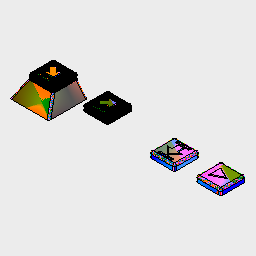
keycaps_debugsymbols_v2 (Autodesk Fusion 360 design; units mm, degrees)
Autodesk Fusion 360 part; units mm, degrees
note: some values were not read from the file. Chosen so that the rebuilt part matches the saved one: which sketch regions a step uses; that a step has no effect.
mesh "Netz1" [no effect]
sketch "Skizze1" plane through (5.433, 7.5669, 0.0261) normal (0, 0, 1) x (1, 0, 0)
  line L0 (-3.1492, -9.717) -> (-7.3992, -9.717) construction
  line L1 (-7.3992, -9.717) -> (-7.3992, -5.467) construction
  line L2 (-7.3992, -5.467) -> (-3.1492, -5.467) construction
  line L3 (-3.1492, -5.467) -> (-3.1492, -9.717) construction
  line L4 (-3.1492, -9.717) -> (-7.3992, -5.467) construction
  line L5 (-7.3992, -9.717) -> (-3.1492, -5.467) construction
  circle A0 centre (-5.2742, -7.592) radius 3.0052
  line L6 (-4.6092, -5.467) -> (-5.9392, -5.467)
  line L7 (-5.9392, -9.717) -> (-4.6092, -9.717)
  line L8 (-4.6092, -5.467) -> (-5.9392, -9.717) construction
  line L9 (-5.9392, -5.467) -> (-4.6092, -9.717) construction
  line L10 (-7.3992, -8.337) -> (-7.3992, -6.847)
  line L11 (-3.1492, -6.847) -> (-3.1492, -8.337)
  line L12 (-3.1492, -8.337) -> (-7.3992, -6.847) construction
  line L13 (-7.3992, -8.337) -> (-3.1492, -6.847) construction
  line L14 (-5.9392, -5.467) -> (-5.9392, -6.847)
  line L15 (-5.9392, -8.337) -> (-5.9392, -9.717)
  line L16 (-3.1492, -8.337) -> (-4.6092, -8.337)
  line L17 (-5.9392, -8.337) -> (-7.3992, -8.337)
  line L18 (-4.6092, -9.717) -> (-4.6092, -8.337)
  line L19 (-4.6092, -6.847) -> (-4.6092, -5.467)
  line L20 (-7.3992, -6.847) -> (-5.9392, -6.847)
  line L21 (-4.6092, -6.847) -> (-3.1492, -6.847)
  line L22 (3.0758, 0.758) -> (-13.6242, 0.758)
  line L23 (-13.6242, 0.758) -> (-13.6242, -15.942)
  line L24 (-13.6242, -15.942) -> (3.0758, -15.942)
  line L25 (3.0758, -15.942) -> (3.0758, 0.758)
  line L26 (3.0758, 0.758) -> (-13.6242, -15.942) construction
  line L27 (-13.6242, 0.758) -> (3.0758, -15.942) construction
  line L28 (4.0758, -16.942) -> (4.0758, 1.758)
  line L29 (4.0758, 1.758) -> (-14.6242, 1.758)
  line L30 (-14.6242, 1.758) -> (-14.6242, -16.942)
  line L31 (-14.6242, -16.942) -> (4.0758, -16.942)
  point P0 (-5.2742, -7.592)
  point P1 (-5.2742, -7.592)
  point P2 (-5.2742, -7.592)
  point P3 (-5.2742, -7.592)
  dimension "d1" = 4.25
  dimension "d2" = 4.25
  dimension "d3" = 1.33
  dimension "d4" = 1.49
  dimension "d10" = 16.7
  dimension "d11" = 16.7
  dimension "d12" = 1
  measures "d1" distance of L1.end L2.end
  measures "d2" distance of L0.end L1.end
  measures "d3" distance of L7.start L7.end
  measures "d4" distance of L10.start L10.end
  measures "d10" distance of L22.end L23.end
  measures "d11" distance of L23.end L24.end
ref_plane "Arbeitsebene1" through (0.1588, -0.0251, 7.0261) normal (0, 0, 1) x (1, 0, 0)
sketch "Skizze2" plane through (0, 0, 7.0261) normal (0, 0, 1) x (-1, 0, 0)
  line L0 (-5.1588, 3.0132) -> (4.8412, 3.0132)
  line L1 (4.8412, 3.0132) -> (4.8412, -6.9868)
  line L2 (4.8412, -6.9868) -> (-5.1588, -6.9868)
  line L3 (-5.1588, -6.9868) -> (-5.1588, 3.0132)
  line L4 (-5.1588, 3.0132) -> (4.8412, -6.9868) construction
  line L5 (4.8412, 3.0132) -> (-5.1588, -6.9868) construction
  line L6 (4.5912, 2.7632) -> (4.5912, -6.7368)
  line L7 (4.5912, -6.7368) -> (-4.9088, -6.7368)
  line L8 (-4.9088, -6.7368) -> (-4.9088, 2.7632)
  line L9 (-4.9088, 2.7632) -> (4.5912, 2.7632)
  line L10 (-6.1588, -7.9868) -> (-6.1588, 4.0132)
  line L11 (-6.1588, 4.0132) -> (5.8412, 4.0132)
  line L12 (5.8412, 4.0132) -> (5.8412, -7.9868)
  line L13 (5.8412, -7.9868) -> (-6.1588, -7.9868)
  point P0 (-0.1588, 0.0251)
  point P1 (-0.1588, 0.0251)
  dimension "d45" = 10
  dimension "d46" = 10
  dimension "d49" = 1
  dimension "d55" = 0.25
  measures "d45" distance of L1.end L2.end
  measures "d46" distance of L0.end L1.end
  measures "d55" distance of L0 L9
sketch "Skizze6" plane through (0, 0, 0) normal (1, 0, 0) x (0, 1, 0)
  spline S0 degree 5 poles (-4.0132, 7.0261) (-4.2644, 6.6286) (-4.7693, 5.9002) (-5.534, 5.0076) (-6.5555, 4.1355) (-7.7576, 3.2091) (-8.5695, 2.2707) (-9.0371, 1.2841) (-9.2748, 0.4713) (-9.3751, 0.0261) knots 0 0 0 0 0 0 0.2 0.4 0.6 0.8 1 1 1 1 1 1
  line L0 (-9.1428, 1.0572) -> (-9.6075, -1.005)
  line L1 (-3.4059, 7.9871) -> (-4.6204, 6.0651)
  line L2 (-4.0132, 7.0261) -> (7.9868, 7.0261)
  point P0 (9.3249, 0.0261)
  point P1 (6.7368, 7.0261)
  point P2 (-2.7632, 7.0261)
  point P3 (-9.3751, 0.0261)
  point P4 (-4.0132, 7.0261)
loft "Erhebung1" add profiles "Skizze1", "Skizze2" section 1 contours A0 | L6 L7 L10 L11 L14 L15 L16 L17 L18 L19 L20 L21 | L22 L23 L24 L25 | L28 L29 L30 L31 section 2 contours L0 L1 L2 L3 | L10 L11 L12 L13 makes body 1
shell "Schale1" thickness 1 removed faces 1 at (-2.9579, 3.0916, 0.0261) on bodies 1
extrude "Extrusion5" add sketch "Skizze2" along normal blind 1 contours L0 L1 L2 L3 | L6 L7 L8 L9 bodies 1
extrude "Extrusion4" add sketch "Skizze2" along normal blind 1.25 contours L0 L1 L2 L3 | L6 L7 L8 L9 bodies 1
extrude "Extrusion1" add sketch "Skizze1" along normal blind 7 contours A0 bodies 1
chamfer "Fase1" distance 2.02 distance2 0.25 1 edges at (-2.6431, -1.1118, 0.0261) measured on face at (3.149, 0.2741, 4.0261) on bodies 1
chamfer "Fase2" distance 1.5 distance2 0.25 12 edges at (0.8238, -1.4601, 0.0261) (0.1588, -2.1501, 0.0261) (-0.5062, -1.4601, 0.0261) (-1.2362, -0.7701, 0.0261) (-1.9662, -0.0251, 0.0261) (-1.2362, 0.7199, 0.0261) (-0.5062, 1.4099, 0.0261) (0.1588, 2.0999, 0.0261) (0.8238, 1.4099, 0.0261) (1.5538, 0.7199, 0.0261) (2.2838, -0.0251, 0.0261) (1.5538, -0.7701, 0.0261) measured on face at (0.8238, -1.6901, 2.0261) measured on face at (-0.0629, -2.1501, 2.0261) measured on face at (-0.5062, -1.2301, 2.0261) measured on face at (-0.9929, -0.7701, 2.0261) measured on face at (-1.9662, -0.2734, 2.0261) measured on face at (-1.4796, 0.7199, 2.0261) measured on face at (-0.5062, 1.6399, 2.0261) measured on face at (0.3804, 2.0999, 2.0261) measured on face at (0.8238, 1.1799, 2.0261) measured on face at (1.3104, 0.7199, 2.0261) measured on face at (2.2838, 0.2232, 2.0261) measured on face at (1.3104, -0.7701, 2.0261) on bodies 1
sketch "Skizze3" plane through (26.215, 27.4055, 0) normal (0, 0, 1) x (1, 0, 0) in component "Symbol1"
  line L0 (3.4862, -25.3196) -> (3.4862, -15.3196)
  line L1 (13.4862, -25.3196) -> (3.4862, -15.3196) construction
  line L2 (13.4862, -25.3196) -> (3.4862, -25.3196)
  line L3 (3.4862, -25.3196) -> (13.4862, -15.3196) construction
  line L4 (13.4862, -15.3196) -> (13.4862, -25.3196)
  line L5 (3.4862, -15.3196) -> (13.4862, -15.3196)
  line L6 (11.4862, -24.7196) -> (8.4862, -24.7196)
  line L7 (5.4862, -19.0653) -> (6.3592, -18.1926)
  line L8 (7.6124, -21.1934) -> (6.3498, -22.4561)
  line L9 (10.6227, -22.4561) -> (6.3498, -22.4561)
  line L10 (8.4862, -24.2196) -> (5.4862, -24.2196)
  line L11 (9.3601, -19.4458) -> (10.6227, -18.1831)
  line L12 (11.4862, -24.2196) -> (11.4862, -24.7196)
  line L13 (5.4862, -19.0653) -> (7.6124, -21.1934)
  line L14 (8.4862, -24.2196) -> (11.4862, -24.2196)
  line L15 (7.232, -17.3196) -> (9.3601, -19.4458)
  line L16 (9.36, -19.0216) -> (7.2319, -16.8954)
  line L17 (8.4862, -23.9196) -> (5.1862, -23.9196)
  line L18 (6.1471, -17.9805) -> (5.062, -19.0652)
  line L19 (10.9227, -22.7561) -> (10.9227, -17.4589)
  line L20 (10.9227, -17.4589) -> (9.36, -19.0216)
  line L21 (8.4862, -23.9196) -> (11.7862, -23.9196)
  line L22 (11.7862, -23.9196) -> (11.7862, -25.0196)
  line L23 (11.7862, -25.0196) -> (8.4862, -25.0196)
  line L24 (5.1862, -25.0196) -> (8.4862, -25.0196)
  line L25 (5.4862, -24.7196) -> (8.4862, -24.7196)
  line L26 (7.232, -17.3196) -> (6.3592, -18.1926)
  line L27 (5.6255, -22.7561) -> (10.9227, -22.7561)
  line L28 (5.4862, -24.2196) -> (5.4862, -24.7196)
  line L29 (10.6227, -22.4561) -> (10.6227, -18.1831)
  line L30 (5.062, -19.0652) -> (7.1882, -21.1933)
  line L31 (7.2319, -16.8954) -> (6.1471, -17.9805)
  line L32 (7.1882, -21.1933) -> (5.6255, -22.7561)
  line L33 (5.1862, -23.9196) -> (5.1862, -25.0196)
  line L34 (3.3362, -25.4696) -> (3.3362, -15.1696)
  line L35 (3.3362, -15.1696) -> (13.6362, -15.1696)
  line L36 (13.6362, -15.1696) -> (13.6362, -25.4696)
  line L37 (13.6362, -25.4696) -> (3.3362, -25.4696)
  line L38 (2.4362, -26.3696) -> (2.4362, -14.2696)
  line L39 (2.4362, -14.2696) -> (14.5362, -14.2696)
  line L40 (14.5362, -14.2696) -> (14.5362, -26.3696)
  line L41 (14.5362, -26.3696) -> (2.4362, -26.3696)
  dimension "d36" = 0.15
  dimension "d40" = 1.05
  dimension "d43" = 10
  dimension "d44" = 10
  measures "d43" distance of L0.end L3.end
  measures "d44" distance of L0.start L0.end
extrude "Extrusion1'" add sketch "Skizze3" along normal blind 0.5 separate body contours L0 L2 L4 L5 | L6 L10 L12 L14 L25 L28 | L7 L8 L9 L11 L13 L15 L26 L29 | L16 L18 L19 L20 L27 L30 L31 L32 | L17 L21 L22 L23 L24 L33 makes body 2 in component "Symbol1"
extrude "Extrusion2" add sketch "Skizze3" along normal blind 1.5 contours L6 L10 L12 L14 L25 L28 | L7 L8 L9 L11 L13 L15 L26 L29 bodies 2 in component "Symbol1"
extrude "Extrusion3" add sketch "Skizze3" along normal blind 0.75 from surface at 0.5 separate body contours L0 L2 L4 L5 | L34 L35 L36 L37 makes body 3 in component "Symbol1"
extrude "Extrusion4'" add sketch "Skizze3" along normal blind 1.25 contours L38 L39 L40 L41 bodies 3 in component "Symbol1"
extrude "Extrusion5'" add sketch "Skizze3" against normal blind 1.5 contours L38 L39 L40 L41 bodies 3 in component "Symbol1"
sketch "Skizze4" plane through (0, 0, 0) normal (0, 0, 1) x (1, 0, 0) in component "Symbol2"
  line L0 (53.1287, 3.5501) -> (56.4287, 3.5501)
  line L1 (56.1287, 11.0501) -> (56.1287, 11.5501)
  line L2 (53.1287, 3.2501) -> (56.1287, 3.2501)
  line L3 (56.4287, 11.8501) -> (56.4287, 10.7501)
  line L4 (50.1287, 11.0501) -> (50.1287, 11.5501)
  line L5 (53.1287, 3.7258) -> (56.853, 7.4501)
  line L6 (53.1287, 4.1501) -> (56.1287, 7.1501)
  line L7 (53.1287, 11.0501) -> (56.1287, 11.0501)
  line L8 (56.1287, 11.5501) -> (53.1287, 11.5501)
  line L9 (53.1287, 2.4501) -> (49.8287, 2.4501)
  line L10 (54.6287, 7.4501) -> (54.6287, 10.4501)
  line L11 (49.8287, 11.8501) -> (53.1287, 11.8501)
  line L12 (56.1287, 2.7501) -> (53.1287, 2.7501)
  line L13 (54.6287, 10.4501) -> (53.1287, 10.4501)
  line L14 (51.9287, 7.1501) -> (50.1287, 7.1501)
  line L15 (49.8287, 3.5501) -> (53.1287, 3.5501)
  line L16 (53.1287, 3.2501) -> (50.1287, 3.2501)
  line L17 (50.1287, 11.5501) -> (53.1287, 11.5501)
  line L18 (53.1287, 4.1501) -> (50.1287, 7.1501)
  line L19 (49.4045, 7.4501) -> (53.1287, 3.7258)
  line L20 (56.1287, 3.2501) -> (56.1287, 2.7501)
  line L21 (50.1287, 3.2501) -> (50.1287, 2.7501)
  line L22 (51.6287, 7.4501) -> (49.4045, 7.4501)
  line L23 (54.3287, 7.1501) -> (56.1287, 7.1501)
  line L24 (53.1287, 11.0501) -> (50.1287, 11.0501)
  line L25 (51.9287, 10.1501) -> (53.1287, 10.1501)
  line L26 (56.4287, 10.7501) -> (53.1287, 10.7501)
  line L27 (48.1287, 12.1501) -> (58.1287, 12.1501)
  line L28 (58.1287, 12.1501) -> (58.1287, 2.1501)
  line L29 (48.1287, 2.1501) -> (58.1287, 12.1501) construction
  line L30 (49.8287, 10.7501) -> (49.8287, 11.8501)
  line L31 (58.1287, 2.1501) -> (48.1287, 12.1501) construction
  line L32 (54.3287, 10.1501) -> (54.3287, 7.1501)
  line L33 (56.4287, 3.5501) -> (56.4287, 2.4501)
  line L34 (50.1287, 2.7501) -> (53.1287, 2.7501)
  line L35 (51.6287, 10.4501) -> (51.6287, 7.4501)
  line L36 (49.8287, 2.4501) -> (49.8287, 3.5501)
  line L37 (51.9287, 10.1501) -> (51.9287, 7.1501)
  line L38 (58.1287, 2.1501) -> (48.1287, 2.1501)
  line L39 (53.1287, 11.8501) -> (56.4287, 11.8501)
  line L40 (53.1287, 10.7501) -> (49.8287, 10.7501)
  line L41 (53.1287, 10.4501) -> (51.6287, 10.4501)
  line L42 (56.853, 7.4501) -> (54.6287, 7.4501)
  line L43 (54.3287, 10.1501) -> (53.1287, 10.1501)
  line L44 (48.1287, 2.1501) -> (48.1287, 12.1501)
  line L45 (56.4287, 2.4501) -> (53.1287, 2.4501)
  line L46 (47.9787, 2.0001) -> (47.9787, 12.3001)
  line L47 (47.9787, 12.3001) -> (58.2787, 12.3001)
  line L48 (58.2787, 12.3001) -> (58.2787, 2.0001)
  line L49 (58.2787, 2.0001) -> (47.9787, 2.0001)
  line L50 (47.0787, 1.1001) -> (47.0787, 13.2001)
  line L51 (47.0787, 13.2001) -> (59.1787, 13.2001)
  line L52 (59.1787, 13.2001) -> (59.1787, 1.1001)
  line L53 (59.1787, 1.1001) -> (47.0787, 1.1001)
  dimension "d72" = 0.15
  dimension "d73" = 1.05
extrude "Extrusion1''" add sketch "Skizze4" along normal blind 0.5 separate body contours L0 L9 L15 L33 L36 L45 | L1 L4 L7 L8 L17 L24 | L2 L12 L16 L20 L21 L34 | L3 L11 L26 L30 L39 L40 | L5 L10 L13 L19 L22 L35 L41 L42 | L6 L14 L18 L23 L25 L32 L37 L43 | L27 L28 L38 L44 makes body 4 in component "Symbol2"
extrude "Extrusion2'" add sketch "Skizze4" along normal blind 1.5 contours L1 L4 L7 L8 L17 L24 | L2 L12 L16 L20 L21 L34 | L6 L14 L18 L23 L25 L32 L37 L43 bodies 4 in component "Symbol2"
extrude "Extrusion3'" add sketch "Skizze4" along normal blind 0.75 from surface at 0.5 separate body contours L27 L28 L38 L44 | L46 L47 L48 L49 makes body 5 in component "Symbol2"
extrude "Extrusion4''" add sketch "Skizze4" along normal blind 1.25 contours L50 L51 L52 L53 bodies 5 in component "Symbol2"
extrude "Extrusion5''" add sketch "Skizze4" against normal blind 1.5 contours L50 L51 L52 L53 bodies 5 in component "Symbol2"
fillet "Abrundung2" radius 1 4 edges at (40.7512, 1.0359, -0.125) (28.6512, 1.0359, -0.125) (40.7512, 13.1359, -0.125) (28.6512, 13.1359, -0.125) on bodies 3 in component "Symbol1"
fillet "Abrundung1" radius 1 8 edges at (40.4583, 12.843, 1.25) (34.7012, 13.1359, 1.25) (28.9441, 12.843, 1.25) (28.6512, 7.0859, 1.25) (28.9441, 1.3288, 1.25) (34.7012, 1.0359, 1.25) (40.4583, 1.3288, 1.25) (40.7512, 7.0859, 1.25) on bodies 3 in component "Symbol1"
fillet "Abrundung5" radius 1 4 edges at (-7.5162, -6.6941, 3.5261) (-7.5162, 8.6559, 3.5261) (7.8338, -6.6941, 3.5261) (7.8338, 8.6559, 3.5261) on bodies 1
fillet "Abrundung1'" radius 1 4 edges at (47.0787, 1.1001, -0.125) (47.0787, 13.2001, -0.125) (59.1787, 13.2001, -0.125) (59.1787, 1.1001, -0.125) on bodies 5 in component "Symbol2"
fillet "Abrundung2'" radius 1 8 edges at (47.3716, 12.9072, 1.25) (47.0787, 7.1501, 1.25) (47.3716, 1.393, 1.25) (53.1287, 1.1001, 1.25) (58.8858, 1.393, 1.25) (59.1787, 7.1501, 1.25) (58.8858, 12.9072, 1.25) (53.1287, 13.2001, 1.25) on bodies 5 in component "Symbol2"
sketch "Skizze5" plane through (0, 0, 0) normal (0, 0, 1) x (1, 0, 0) in component "symbol3"
  line L0 (79.313, 3.1314) -> (69.313, 13.1314) construction
  line L1 (79.313, 13.1314) -> (79.313, 3.1314)
  line L2 (71.613, 5.6168) -> (76.6422, 8.1314)
  line L3 (71.613, 10.646) -> (71.613, 5.6168)
  line L4 (79.313, 3.1314) -> (69.313, 3.1314)
  line L5 (76.6422, 8.1314) -> (71.613, 10.646)
  line L6 (69.313, 13.1314) -> (79.313, 13.1314)
  line L7 (69.313, 3.1314) -> (69.313, 13.1314)
  line L8 (71.313, 5.1314) -> (71.313, 11.1314)
  line L9 (71.313, 11.1314) -> (77.313, 8.1314)
  line L10 (77.313, 8.1314) -> (71.313, 5.1314)
  line L11 (69.313, 3.1314) -> (79.313, 13.1314) construction
  line L12 (69.163, 2.9814) -> (69.163, 13.2814)
  line L13 (69.163, 13.2814) -> (79.463, 13.2814)
  line L14 (79.463, 13.2814) -> (79.463, 2.9814)
  line L15 (79.463, 2.9814) -> (69.163, 2.9814)
  line L16 (68.263, 2.0814) -> (68.263, 14.1814)
  line L17 (68.263, 14.1814) -> (80.363, 14.1814)
  line L18 (80.363, 14.1814) -> (80.363, 2.0814)
  line L19 (80.363, 2.0814) -> (68.263, 2.0814)
  dimension "d88" = 0.15
  dimension "d89" = 1.05
extrude "Extrusion1'''" add sketch "Skizze5" along normal blind 0.5 separate body contours L1 L4 L6 L7 | L2 L3 L5 | L8 L9 L10 makes body 6 in component "symbol3"
extrude "Extrusion2''" add sketch "Skizze5" along normal blind 1.5 contours L2 L3 L5 bodies 6 in component "symbol3"
extrude "Extrusion4'''" add sketch "Skizze5" along normal blind 0.75 from surface at 0.5 separate body contours L1 L4 L6 L7 | L12 L13 L14 L15 makes body 7 in component "symbol3"
extrude "Extrusion5'''" add sketch "Skizze5" along normal blind 1.25 contours L16 L17 L18 L19 bodies 7 in component "symbol3"
extrude "Extrusion6" add sketch "Skizze5" against normal blind 1.5 contours L16 L17 L18 L19 bodies 7 in component "symbol3"
fillet "Abrundung1''" radius 1 4 edges at (68.263, 2.0814, -0.125) (80.363, 2.0814, -0.125) (80.363, 14.1814, -0.125) (68.263, 14.1814, -0.125) on bodies 7 in component "symbol3"
fillet "Abrundung2''" radius 1 8 edges at (68.5559, 2.3743, 1.25) (74.313, 2.0814, 1.25) (80.0701, 2.3743, 1.25) (80.363, 8.1314, 1.25) (80.0701, 13.8885, 1.25) (74.313, 14.1814, 1.25) (68.5559, 13.8885, 1.25) (68.263, 8.1314, 1.25) on bodies 7 in component "symbol3"
sketch "Skizze3 (2)" plane through (26.215, 27.4055, 0) normal (0, 0, 1) x (1, 0, 0) in component "Symbol4"
  line L0 (3.4862, -25.3196) -> (3.4862, -15.3196)
  line L1 (13.4862, -25.3196) -> (3.4862, -15.3196) construction
  line L2 (13.4862, -25.3196) -> (3.4862, -25.3196)
  line L3 (3.4862, -25.3196) -> (13.4862, -15.3196) construction
  line L4 (13.4862, -15.3196) -> (13.4862, -25.3196)
  line L5 (3.4862, -15.3196) -> (13.4862, -15.3196)
  line L6 (11.4862, -24.7196) -> (8.4862, -24.7196)
  line L7 (7.232, -22.9731) -> (6.3592, -22.1001)
  line L8 (9.3601, -20.8469) -> (10.6227, -22.1096)
  line L9 (10.6227, -17.8366) -> (10.6227, -22.1096)
  line L10 (8.4862, -24.2196) -> (5.4862, -24.2196)
  line L11 (7.6124, -19.0992) -> (6.3498, -17.8366)
  line L12 (11.4862, -24.2196) -> (11.4862, -24.7196)
  line L13 (7.232, -22.9731) -> (9.3601, -20.8469)
  line L14 (8.4862, -24.2196) -> (11.4862, -24.2196)
  line L15 (5.4862, -21.2273) -> (7.6124, -19.0992)
  line L16 (7.1882, -19.0993) -> (5.062, -21.2275)
  line L17 (8.4862, -23.9196) -> (5.1862, -23.9196)
  line L18 (6.1471, -22.3122) -> (7.2319, -23.3973)
  line L19 (10.9227, -17.5366) -> (5.6255, -17.5366)
  line L20 (5.6255, -17.5366) -> (7.1882, -19.0993)
  line L21 (8.4862, -23.9196) -> (11.7862, -23.9196)
  line L22 (11.7862, -23.9196) -> (11.7862, -25.0196)
  line L23 (11.7862, -25.0196) -> (8.4862, -25.0196)
  line L24 (5.1862, -25.0196) -> (8.4862, -25.0196)
  line L25 (5.4862, -24.7196) -> (8.4862, -24.7196)
  line L26 (5.4862, -21.2273) -> (6.3592, -22.1001)
  line L27 (10.9227, -22.8338) -> (10.9227, -17.5366)
  line L28 (5.4862, -24.2196) -> (5.4862, -24.7196)
  line L29 (10.6227, -17.8366) -> (6.3498, -17.8366)
  line L30 (7.2319, -23.3973) -> (9.36, -21.2711)
  line L31 (5.062, -21.2275) -> (6.1471, -22.3122)
  line L32 (9.36, -21.2711) -> (10.9227, -22.8338)
  line L33 (5.1862, -23.9196) -> (5.1862, -25.0196)
  line L34 (3.3362, -25.4696) -> (3.3362, -15.1696)
  line L35 (3.3362, -15.1696) -> (13.6362, -15.1696)
  line L36 (13.6362, -15.1696) -> (13.6362, -25.4696)
  line L37 (13.6362, -25.4696) -> (3.3362, -25.4696)
  line L38 (2.4362, -26.3696) -> (2.4362, -14.2696)
  line L39 (2.4362, -14.2696) -> (14.5362, -14.2696)
  line L40 (14.5362, -14.2696) -> (14.5362, -26.3696)
  line L41 (14.5362, -26.3696) -> (2.4362, -26.3696)
  dimension "d36_1" = 0.15
  dimension "d40_1" = 1.05
  dimension "d43_1" = 10
  dimension "d44_1" = 10
  measures "d43_1" distance of L0.end L3.end
  measures "d44_1" distance of L0.start L0.end
extrude "Extrusion1''''" add sketch "Skizze3 (2)" along normal blind 0.5 separate body contours L0 L2 L4 L5 | L6 L10 L12 L14 L25 L28 | L7 L8 L9 L11 L13 L15 L26 L29 | L16 L18 L19 L20 L27 L30 L31 L32 | L17 L21 L22 L23 L24 L33 makes body 8 in component "Symbol4"
extrude "Extrusion2'''" add sketch "Skizze3 (2)" along normal blind 1.5 contours L6 L10 L12 L14 L25 L28 | L7 L8 L9 L11 L13 L15 L26 L29 bodies 8 in component "Symbol4"
extrude "Extrusion3''" add sketch "Skizze3 (2)" along normal blind 0.75 from surface at 0.5 separate body contours L0 L2 L4 L5 | L34 L35 L36 L37 makes body 9 in component "Symbol4"
extrude "Extrusion4''''" add sketch "Skizze3 (2)" along normal blind 1.25 contours L38 L39 L40 L41 bodies 9 in component "Symbol4"
extrude "Extrusion5''''" add sketch "Skizze3 (2)" against normal blind 1.5 contours L38 L39 L40 L41 bodies 9 in component "Symbol4"
fillet "Abrundung2'''" radius 1 4 edges at (40.7512, 1.0359, -0.125) (28.6512, 1.0359, -0.125) (40.7512, 13.1359, -0.125) (28.6512, 13.1359, -0.125) on bodies 9 in component "Symbol4"
fillet "Abrundung1'''" radius 1 8 edges at (40.4583, 12.843, 1.25) (34.7012, 13.1359, 1.25) (28.9441, 12.843, 1.25) (28.6512, 7.0859, 1.25) (28.9441, 1.3288, 1.25) (34.7012, 1.0359, 1.25) (40.4583, 1.3288, 1.25) (40.7512, 7.0859, 1.25) on bodies 9 in component "Symbol4"
component "Symbol1" placed x (1, 0, 0) y (0, 1, 0) z (0, 0, 1) at (-34.4925, -5.049, 8.5261)
component "Symbol2" placed x (1, 0, 0) y (0, 1, 0) z (0, 0, 1) at (0, 0, 0)
component "symbol3" placed x (1, 0, 0) y (0, 1, 0) z (0, 0, 1) at (0, 0, 0)
component "Symbol4" placed x (1, 0, 0) y (0, 1, 0) z (0, 0, 1) at (-8.5012, -5.049, 8.5261)
equation "d1 = 4 mm + pcf"
equation "d2 = 4 mm + pcf"
equation "d3 = 1.08 mm + pcf"
equation "d4 = 1.24 mm + pcf"
equation "pcf = 0.25 mm"
equation "d12 = wand"
equation "wand = 1 mm"
equation "radius = 1.8 mm"
equation "d25 = pcf"
equation "d27 = pcf"
equation "d28 = symboldicke / 2"
equation "d30 = symboldicke * 1.5"
equation "d33 = symboldicke - pcf"
equation "symboldicke = 1 mm"
equation "d36 = fest"
equation "nozzle = 0.4 mm"
equation "d40 = pcf + nozzle * 2"
equation "d49 = wand"
equation "d50 = 1 mm + pcf"
equation "d52 = wand"
equation "d55 = pcf"
equation "d72 = fest"
equation "d73 = pcf + nozzle * 2"
equation "d74 = symboldicke / 2"
equation "d76 = symboldicke * 1.5"
equation "d79 = symboldicke - pcf"
equation "fest = pcf * 0.6"
equation "d88 = fest"
equation "d89 = pcf + nozzle * 2"
equation "d90 = symboldicke / 2"
equation "d92 = symboldicke * 1.5"
equation "d97 = symboldicke - pcf"
equation "d28_1 = symboldicke / 2"
equation "d30_1 = symboldicke * 1.5"
equation "d33_1 = symboldicke - pcf"
equation "d36_1 = fest"
equation "d40_1 = pcf + nozzle * 2"
named bodies: "inner-s1", "clip-s1", "base", "inner-s2", "clip-s2", "inner-s3", "clip-s3", "inner-s4", "clip-s4"
